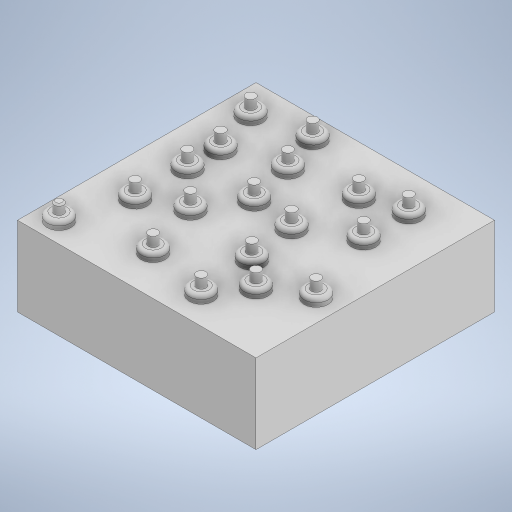
# Autodesk Inventor part: 草圖驅動式
Saved by Autodesk Inventor 2024.2 (Build 282272000, 272)
## iProperties
Created: 2024-05-02
Part Number: 草圖驅動式
Material: 一般
Document SubType Name: Modeling
Designer: User
Density: 1 g/cm^3
Appearance: 預設
Author: User
Autodesk Inventor part; units mm, degrees
ref_plane "YZ Plane" through (0, 0, 0) normal (1, 0, 0) x (0, 1, 0)
ref_plane "XZ Plane" through (0, 0, 0) normal (0, 1, 0) x (-1, 0, 0)
ref_plane "XY Plane" through (0, 0, 0) normal (0, 0, 1) x (1, 0, 0)
sketch "草圖1" plane through (0, 0, 0) normal (0, 1, 0) x (-1, 0, 0)
  line L0 (15, -15) -> (-15, -15)
  line L1 (-15, -15) -> (-15, 15)
  line L2 (-15, 15) -> (15, 15)
  line L3 (15, 15) -> (15, -15)
  line L4 (15, -15) -> (-15, 15) construction
  line L5 (-15, -15) -> (15, 15) construction
  point P0 (0, 0)
  dimension "d0" = 30
  dimension "d1" = 30
  constraints: 12 end point, 2 midpoint, 2 parallel, 1 horizontal, 1 perpendicular
  measures "d0" distance of L1.end L2.end
  measures "d1" distance of L0.end L1.end
extrude "擠出1" add sketch "草圖1" along normal blind 10
sketch "草圖2" plane through (0, 10, 0) normal (0, 1, 0) x (1, 0, 0)
  circle A0 centre (-12.3284, -12.4598) radius 1.5
  point P0 (0, 0)
  dimension "d4" = 3
  constraints: 1 centre point
  measures "d4" diameter of A0
extrude "擠出2" add sketch "草圖2" along normal blind 1
sketch "草圖3" plane through (-12.3284, 11, 12.4598) normal (0, 1, 0) x (1, 0, 0)
  circle A0 centre (0, 0) radius 0.6
  point P0 (12.3284, 12.4598)
  dimension "d7" = 1.2
  constraints: 1 centre point
  measures "d7" diameter of A0
extrude "擠出3" add sketch "草圖3" along normal blind 1.2
fillet "圓角1" radius 0.5 1 edges at (-13.8284, 11, 12.4598)
chamfer "倒角1" distance 0.2 angle 45 1 edges at (-12.9284, 12.2, 12.4598)
pattern_sketch "草圖驅動式陣列1" of "圓角1", "擠出3", "擠出2" from (-12.3284, 10, 12.4598) copies at (-11.6916, 10, -11.0106) at (-5.1837, 10, -12.297) at (-3.5188, 10, -7.5296) at (8.9674, 10, -10.2538) at (8.9674, 10, -4.5783) at (4.1242, 10, -8.816) at (-5.1837, 10, 3.0648) at (-9.8755, 10, 5.335) at (-9.8755, 10, -1.2486) at (-9.8755, 10, -5.4107) at (7.5296, 10, 7.5296) at (4.1242, 10, 4.654) at (-2.9135, 10, 10.0268) at (4.654, 10, 11.5403) at (12.2214, 10, 4.654) at (3.2161, 10, -1.2486) at (-2.1567, 10, -1.9297)
sketch "草圖4" plane through (0, 10, 0) normal (0, 1, 0) x (1, 0, 0)
  point P0 (0, 0)
  point P1 (-11.6916, 11.0106)
  point P2 (-5.1837, 12.297)
  point P3 (-3.5188, 7.5296)
  point P4 (8.9674, 10.2538)
  point P5 (8.9674, 4.5783)
  point P6 (4.1242, 8.816)
  point P7 (-5.1837, -3.0648)
  point P8 (-9.8755, -5.335)
  point P9 (-9.8755, 1.2486)
  point P10 (-9.8755, 5.4107)
  point P11 (7.5296, -7.5296)
  point P12 (4.1242, -4.654)
  point P13 (-2.9135, -10.0268)
  point P14 (4.654, -11.5403)
  point P15 (12.2214, -4.654)
  point P16 (3.2161, 1.2486)
  point P17 (-2.1567, 1.9297)
